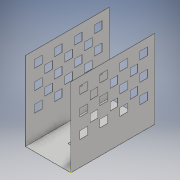
# Autodesk Inventor part: 3sqr x 1sqr x 3sqr metal connector
Saved by Autodesk Inventor 2018 (Build 220112000, 112)
## iProperties
Created: 2018-11-08
Part Number: 3sqr x 1sqr x 3sqr metal connector
Material: Generic
Document SubType Name: Modeling
Designer: USER
Density: 1 g/cm^3
Appearance: Default
Author: USER
Autodesk Inventor part; units mm, degrees
ref_plane "YZ Plane" through (0, 0, 0) normal (1, 0, 0) x (0, 1, 0)
ref_plane "XZ Plane" through (0, 0, 0) normal (0, 1, 0) x (-1, 0, 0)
ref_plane "XY Plane" through (0, 0, 0) normal (0, 0, 1) x (1, 0, 0)
sketch "Sketch1" plane through (0, 0, 0) normal (1, 0, 0) x (0, 1, 0)
  line L0 (0, 0) -> (47, 0)
  line L1 (47, 0) -> (47, -50)
  line L2 (47, -50) -> (0, -50)
  line L3 (0, -50) -> (0, 0)
  dimension "d0" = 47
  dimension "d1" = 50
  constraints: 8 end point, 2 parallel, 1 horizontal, 1 perpendicular
  measures "d0" distance of L1.end L2.end
  measures "d1" distance of L0.end L1.end
sketch "Sketch2" plane through (0, 0, 0) normal (0, 1, 0) x (-1, 0, 0)
  line L0 (0, 0) -> (-27, 0)
  line L1 (-27, 0) -> (-27, -50)
  line L2 (-27, -50) -> (0, -50)
  line L3 (0, -50) -> (0, 0)
  dimension "d2" = 27
  dimension "d3" = 50
  constraints: 8 end point, 2 parallel, 1 horizontal, 1 perpendicular
  measures "d2" distance of L2.end L1.end
  measures "d3" distance of L1.end L0.end
extrude "Extrusion1" add sketch "Sketch1" against normal blind 0.1
extrude "Extrusion2" add sketch "Sketch2" along normal blind 0.1 separate body
sketch "Sketch3" plane through (27, 0, 0) normal (1, 0, 0) x (0, 0, -1)
  point P0 (0, 0)
sketch "Sketch4" plane through (27, 0, 0) normal (1, 0, 0) x (0, 0, -1)
  line L0 (0, 0) -> (50, 0)
  line L1 (50, 0) -> (50, 47)
  line L2 (50, 47) -> (0, 47)
  line L3 (0, 47) -> (0, 0)
  dimension "d8" = 50
  dimension "d9" = 47
  constraints: 8 end point, 2 parallel, 1 horizontal, 1 perpendicular
  measures "d8" distance of L2.end L1.end
  measures "d9" distance of L1.end L0.end
extrude "Extrusion3" add sketch "Sketch4" along normal blind 0.1 separate body
sketch "Sketch5" plane through (0, 0.1, 0) normal (0, 1, 0) x (1, 0, 0)
  line L0 (11.0853, 42.5245) -> (15.6573, 42.5245)
  line L1 (15.6573, 42.5245) -> (15.6573, 37.9525)
  line L2 (15.6573, 37.9525) -> (11.0853, 37.9525)
  line L3 (11.0853, 37.9525) -> (11.0853, 42.5245)
  line L4 (11.0853, 30.6245) -> (15.6573, 30.6245)
  line L5 (15.6573, 30.6245) -> (15.6573, 26.0525)
  line L6 (15.6573, 26.0525) -> (11.0853, 26.0525)
  line L7 (11.0853, 26.0525) -> (11.0853, 30.6245)
  line L8 (11.0853, 18.7245) -> (15.6573, 18.7245)
  line L9 (15.6573, 18.7245) -> (15.6573, 14.1525)
  line L10 (15.6573, 14.1525) -> (11.0853, 14.1525)
  line L11 (11.0853, 14.1525) -> (11.0853, 18.7245)
  point P0 (0, 0)
  dimension "d12" = 4.572
  dimension "d13" = 4.572
  dimension "d16" = 11.9
  constraints: 24 end point, 2 parallel, 1 collinear, 1 horizontal, 1 perpendicular, 1 vertical, 15 other
  measures "d12" distance of L1.end L2.end
  measures "d13" distance of L0.end L1.end
  measures "d16" distance of L0.start L4.start
extrude "Extrusion4" cut sketch "Sketch5" against normal through all bodies 2
sketch "Sketch6" plane through (27.1, 0, 0) normal (1, 0, 0) x (0, 0, -1)
  line L0 (45.6917, 42.2916) -> (41.1197, 42.2916)
  line L1 (41.1197, 42.2916) -> (41.1197, 37.7196)
  line L2 (41.1197, 37.7196) -> (45.6917, 37.7196)
  line L3 (45.6917, 37.7196) -> (45.6917, 42.2916)
  line L4 (33.7917, 37.7196) -> (33.7917, 42.2916)
  line L5 (33.7917, 42.2916) -> (29.2197, 42.2916)
  line L6 (29.2197, 42.2916) -> (29.2197, 37.7196)
  line L7 (29.2197, 37.7196) -> (33.7917, 37.7196)
  line L8 (21.8917, 37.7196) -> (21.8917, 42.2916)
  line L9 (21.8917, 42.2916) -> (17.3197, 42.2916)
  line L10 (17.3197, 42.2916) -> (17.3197, 37.7196)
  line L11 (17.3197, 37.7196) -> (21.8917, 37.7196)
  line L12 (9.9917, 37.7196) -> (9.9917, 42.2916)
  line L13 (9.9917, 42.2916) -> (5.4197, 42.2916)
  line L14 (5.4197, 42.2916) -> (5.4197, 37.7196)
  line L15 (5.4197, 37.7196) -> (9.9917, 37.7196)
  line L16 (45.6917, 26.1196) -> (45.6917, 30.6916)
  line L17 (45.6917, 30.6916) -> (41.1197, 30.6916)
  line L18 (41.1197, 30.6916) -> (41.1197, 26.1196)
  line L19 (41.1197, 26.1196) -> (45.6917, 26.1196)
  line L20 (33.7917, 26.1196) -> (33.7917, 30.6916)
  line L21 (33.7917, 30.6916) -> (29.2197, 30.6916)
  line L22 (29.2197, 30.6916) -> (29.2197, 26.1196)
  line L23 (29.2197, 26.1196) -> (33.7917, 26.1196)
  line L24 (21.8917, 26.1196) -> (21.8917, 30.6916)
  line L25 (21.8917, 30.6916) -> (17.3197, 30.6916)
  line L26 (17.3197, 30.6916) -> (17.3197, 26.1196)
  line L27 (17.3197, 26.1196) -> (21.8917, 26.1196)
  line L28 (9.9917, 26.1196) -> (9.9917, 30.6916)
  line L29 (9.9917, 30.6916) -> (5.4197, 30.6916)
  line L30 (5.4197, 30.6916) -> (5.4197, 26.1196)
  line L31 (5.4197, 26.1196) -> (9.9917, 26.1196)
  line L32 (45.6917, 14.5196) -> (45.6917, 19.0916)
  line L33 (45.6917, 19.0916) -> (41.1197, 19.0916)
  line L34 (41.1197, 19.0916) -> (41.1197, 14.5196)
  line L35 (41.1197, 14.5196) -> (45.6917, 14.5196)
  line L36 (33.7917, 14.5196) -> (33.7917, 19.0916)
  line L37 (33.7917, 19.0916) -> (29.2197, 19.0916)
  line L38 (29.2197, 19.0916) -> (29.2197, 14.5196)
  line L39 (29.2197, 14.5196) -> (33.7917, 14.5196)
  line L40 (21.8917, 14.5196) -> (21.8917, 19.0916)
  line L41 (21.8917, 19.0916) -> (17.3197, 19.0916)
  line L42 (17.3197, 19.0916) -> (17.3197, 14.5196)
  line L43 (17.3197, 14.5196) -> (21.8917, 14.5196)
  line L44 (9.9917, 14.5196) -> (9.9917, 19.0916)
  line L45 (9.9917, 19.0916) -> (5.4197, 19.0916)
  line L46 (5.4197, 19.0916) -> (5.4197, 14.5196)
  line L47 (5.4197, 14.5196) -> (9.9917, 14.5196)
  line L48 (39.8871, 36.4278) -> (35.3151, 36.4278)
  line L49 (35.3151, 36.4278) -> (35.3151, 31.8558)
  line L50 (35.3151, 31.8558) -> (39.8871, 31.8558)
  line L51 (39.8871, 31.8558) -> (39.8871, 36.4278)
  line L52 (39.8871, 20.2558) -> (39.8871, 24.8278)
  line L53 (35.3151, 24.8278) -> (35.3151, 20.2558)
  line L54 (35.3151, 20.2558) -> (39.8871, 20.2558)
  line L55 (39.8871, 24.8278) -> (35.3151, 24.8278)
  line L56 (27.9871, 31.8558) -> (27.9871, 36.4278)
  line L57 (23.4151, 36.4278) -> (23.4151, 31.8558)
  line L58 (23.4151, 31.8558) -> (27.9871, 31.8558)
  line L59 (27.9871, 36.4278) -> (23.4151, 36.4278)
  line L60 (27.9871, 20.2558) -> (27.9871, 24.8278)
  line L61 (23.4151, 24.8278) -> (23.4151, 20.2558)
  line L62 (23.4151, 20.2558) -> (27.9871, 20.2558)
  line L63 (27.9871, 24.8278) -> (23.4151, 24.8278)
  line L64 (16.0871, 31.8558) -> (16.0871, 36.4278)
  line L65 (11.5151, 36.4278) -> (11.5151, 31.8558)
  line L66 (11.5151, 31.8558) -> (16.0871, 31.8558)
  line L67 (16.0871, 36.4278) -> (11.5151, 36.4278)
  line L68 (16.0871, 20.2558) -> (16.0871, 24.8278)
  line L69 (11.5151, 24.8278) -> (11.5151, 20.2558)
  line L70 (11.5151, 20.2558) -> (16.0871, 20.2558)
  line L71 (16.0871, 24.8278) -> (11.5151, 24.8278)
  point P0 (0, 0)
  dimension "d23" = 4.572
  dimension "d24" = 4.572
  dimension "d27" = 11.9
  dimension "d30" = 11.6
  dimension "d33" = 4.572
  dimension "d34" = 4.572
  dimension "d37" = 11.6
  dimension "d40" = 11.9
  constraints: 144 end point, 4 collinear, 4 horizontal, 4 parallel, 2 perpendicular, 2 vertical, 124 other
  measures "d23" distance of L2.end L1.end
  measures "d24" distance of L1.end L0.end
  measures "d27" distance of L2.end L4.start
  measures "d30" distance of L2.end L16.start
  measures "d33" distance of L50.end L49.end
  measures "d34" distance of L49.end L48.end
  measures "d37" distance of L50.end L52.start
  measures "d40" distance of L50.end L56.start
extrude "Extrusion5" cut sketch "Sketch6" against normal through all bodies 3
sketch "Sketch7" plane through (-0.1, 0, 0) normal (-1, 0, 0) x (0, 0, 1)
  line L0 (-41.1197, 37.7196) -> (-41.1197, 42.2916) projected
  line L1 (-45.6917, 37.7196) -> (-41.1197, 37.7196) projected
  line L2 (-41.1197, 42.2916) -> (-45.6917, 42.2916)
  line L3 (-45.6917, 42.2916) -> (-45.6917, 37.7196)
  line L4 (-45.6917, 37.7196) -> (-41.1197, 37.7196)
  line L5 (-41.1197, 37.7196) -> (-41.1197, 42.2916)
  line L6 (-29.2197, 42.2916) -> (-33.7917, 42.2916)
  line L7 (-33.7917, 42.2916) -> (-33.7917, 37.7196)
  line L8 (-33.7917, 37.7196) -> (-29.2197, 37.7196)
  line L9 (-29.2197, 37.7196) -> (-29.2197, 42.2916)
  line L10 (-17.3197, 42.2916) -> (-21.8917, 42.2916)
  line L11 (-21.8917, 42.2916) -> (-21.8917, 37.7196)
  line L12 (-21.8917, 37.7196) -> (-17.3197, 37.7196)
  line L13 (-17.3197, 37.7196) -> (-17.3197, 42.2916)
  line L14 (-5.4197, 42.2916) -> (-9.9917, 42.2916)
  line L15 (-9.9917, 42.2916) -> (-9.9917, 37.7196)
  line L16 (-9.9917, 37.7196) -> (-5.4197, 37.7196)
  line L17 (-5.4197, 37.7196) -> (-5.4197, 42.2916)
  line L18 (-41.1197, 30.6916) -> (-45.6917, 30.6916)
  line L19 (-45.6917, 30.6916) -> (-45.6917, 26.1196)
  line L20 (-45.6917, 26.1196) -> (-41.1197, 26.1196)
  line L21 (-41.1197, 26.1196) -> (-41.1197, 30.6916)
  line L22 (-29.2197, 30.6916) -> (-33.7917, 30.6916)
  line L23 (-33.7917, 30.6916) -> (-33.7917, 26.1196)
  line L24 (-33.7917, 26.1196) -> (-29.2197, 26.1196)
  line L25 (-29.2197, 26.1196) -> (-29.2197, 30.6916)
  line L26 (-17.3197, 30.6916) -> (-21.8917, 30.6916)
  line L27 (-21.8917, 30.6916) -> (-21.8917, 26.1196)
  line L28 (-21.8917, 26.1196) -> (-17.3197, 26.1196)
  line L29 (-17.3197, 26.1196) -> (-17.3197, 30.6916)
  line L30 (-5.4197, 30.6916) -> (-9.9917, 30.6916)
  line L31 (-9.9917, 30.6916) -> (-9.9917, 26.1196)
  line L32 (-9.9917, 26.1196) -> (-5.4197, 26.1196)
  line L33 (-5.4197, 26.1196) -> (-5.4197, 30.6916)
  line L34 (-41.1197, 19.0916) -> (-45.6917, 19.0916)
  line L35 (-45.6917, 19.0916) -> (-45.6917, 14.5196)
  line L36 (-45.6917, 14.5196) -> (-41.1197, 14.5196)
  line L37 (-41.1197, 14.5196) -> (-41.1197, 19.0916)
  line L38 (-29.2197, 19.0916) -> (-33.7917, 19.0916)
  line L39 (-33.7917, 19.0916) -> (-33.7917, 14.5196)
  line L40 (-33.7917, 14.5196) -> (-29.2197, 14.5196)
  line L41 (-29.2197, 14.5196) -> (-29.2197, 19.0916)
  line L42 (-17.3197, 19.0916) -> (-21.8917, 19.0916)
  line L43 (-21.8917, 19.0916) -> (-21.8917, 14.5196)
  line L44 (-21.8917, 14.5196) -> (-17.3197, 14.5196)
  line L45 (-17.3197, 14.5196) -> (-17.3197, 19.0916)
  line L46 (-5.4197, 19.0916) -> (-9.9917, 19.0916)
  line L47 (-9.9917, 19.0916) -> (-9.9917, 14.5196)
  line L48 (-9.9917, 14.5196) -> (-5.4197, 14.5196)
  line L49 (-5.4197, 14.5196) -> (-5.4197, 19.0916)
  line L50 (-35.3151, 31.8558) -> (-35.3151, 36.4278) projected
  line L51 (-39.8871, 36.4278) -> (-39.8871, 31.8558) projected
  line L52 (-35.3151, 36.4278) -> (-39.8871, 36.4278)
  line L53 (-39.8871, 36.4278) -> (-39.8871, 31.8558)
  line L54 (-39.8871, 31.8558) -> (-35.3151, 31.8558)
  line L55 (-35.3151, 31.8558) -> (-35.3151, 36.4278)
  line L56 (-35.3151, 24.8278) -> (-39.8871, 24.8278)
  line L57 (-35.3151, 20.2558) -> (-35.3151, 24.8278)
  line L58 (-39.8871, 20.2558) -> (-35.3151, 20.2558)
  line L59 (-39.8871, 24.8278) -> (-39.8871, 20.2558)
  line L60 (-23.4151, 36.4278) -> (-27.9871, 36.4278)
  line L61 (-23.4151, 31.8558) -> (-23.4151, 36.4278)
  line L62 (-27.9871, 31.8558) -> (-23.4151, 31.8558)
  line L63 (-27.9871, 36.4278) -> (-27.9871, 31.8558)
  line L64 (-23.4151, 24.8278) -> (-27.9871, 24.8278)
  line L65 (-23.4151, 20.2558) -> (-23.4151, 24.8278)
  line L66 (-27.9871, 20.2558) -> (-23.4151, 20.2558)
  line L67 (-27.9871, 24.8278) -> (-27.9871, 20.2558)
  line L68 (-11.5151, 36.4278) -> (-16.0871, 36.4278)
  line L69 (-11.5151, 31.8558) -> (-11.5151, 36.4278)
  line L70 (-16.0871, 31.8558) -> (-11.5151, 31.8558)
  line L71 (-16.0871, 36.4278) -> (-16.0871, 31.8558)
  line L72 (-11.5151, 24.8278) -> (-16.0871, 24.8278)
  line L73 (-11.5151, 20.2558) -> (-11.5151, 24.8278)
  line L74 (-16.0871, 20.2558) -> (-11.5151, 20.2558)
  line L75 (-16.0871, 24.8278) -> (-16.0871, 20.2558)
  point P0 (0, 0)
  dimension "d47" = 11.9
  dimension "d50" = 11.6
  dimension "d55" = 11.6
  dimension "d58" = 11.9
  constraints: 144 end point, 4 horizontal, 4 parallel, 2 collinear, 2 perpendicular, 2 vertical, 126 other
  measures "d47" distance of L0.end L6.start
  measures "d50" distance of L0.end L18.start
  measures "d55" distance of L50.end L56.start
  measures "d58" distance of L50.end L60.start
extrude "Extrusion6" cut sketch "Sketch7" against normal through all bodies 1
body "Solid1"
body "Solid2"
body "Solid3"
